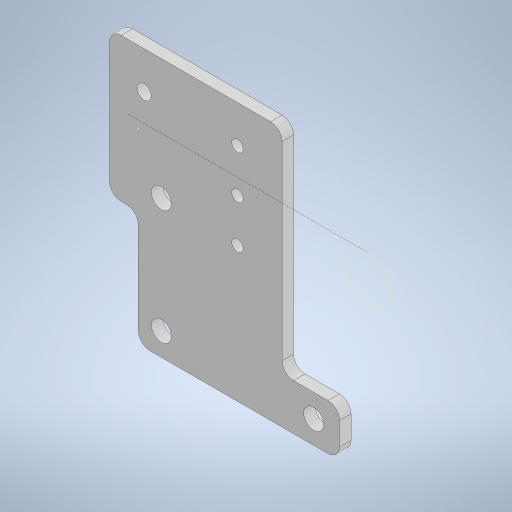
# Autodesk Inventor part: креп_центр_рейки
Saved by Autodesk Inventor 2023.1 (Build 271208000, 208)
## iProperties
Created: 2025-11-24
Part Number: креп_центр_рейки
Material: Типовые
Document SubType Name: Modeling
Designer: DELL
Density: 1 g/cm^3
Appearance: По умолчанию
Author: DELL
Autodesk Inventor part; units mm, degrees
ref_plane "YZ Plane" through (0, 0, 0) normal (1, 0, 0) x (0, 1, 0)
ref_plane "XZ Plane" through (0, 0, 0) normal (0, 1, 0) x (-1, 0, 0)
ref_plane "XY Plane" through (0, 0, 0) normal (0, 0, 1) x (1, 0, 0)
sketch "Эскиз1" plane through (0, 0, 0) normal (0, 0, 1) x (1, 0, 0)
  line L0 (4, 0) -> (50, 0)
  line L1 (70, -4) -> (70, -49)
  line L2 (66, -65) -> (4, -65)
  line L3 (0, -61) -> (0, -4)
  arc A0 (70, -4) -> (66, 0) centre (66, -4) ccw
  arc A1 (66, -65) -> (70, -61) centre (66, -61) ccw
  arc A2 (4, 0) -> (0, -4) centre (4, -4) ccw
  arc A3 (0, -61) -> (4, -65) centre (4, -61) ccw
  line L4 (-10, 25) -> (50, 25)
  line L5 (65, 25) -> (65, -25)
  line L6 (65, -25) -> (-10, -25)
  line L7 (-10, -25) -> (-10, 25)
  line L8 (-10, 25) -> (65, -25) construction
  line L9 (65, 25) -> (-10, -25) construction
  line L10 (70, -49) -> (50, -49)
  line L11 (50, -49) -> (50, 25)
  line L12 (70, -49) -> (70, -61)
  line L13 (65, 0) -> (66, 0)
  line L14 (50, 0) -> (65, 0)
  line L15 (50, 25) -> (65, 25)
  point P0 (0, 0)
  point P1 (70, -65)
  point P2 (70, 0)
  point P3 (27.5, 0)
  point P4 (5, 0)
  point P5 (65, 0)
  point P6 (50, -25)
  point P7 (0, -25)
  dimension "d0" = 70
  dimension "d1" = 65
  dimension "d2" = 4
  dimension "d23" = 75
  dimension "d24" = 50
  dimension "d44" = 20
  dimension "d46" = 16
  dimension "d47" = 5
  dimension "d48" = 25
  constraints: 32 end point, 14 tangent, 10 perpendicular, 8 parallel, 8 point on circle, 7 point on line, 6 horizontal, 4 centre point, 3 equal radius, 3 midpoint
  measures "d0" distance of point (0, 0) point (70, 0)
  measures "d1" distance of point (70, 0) point (70, -65)
  measures "d2" radius of A0
  measures "d23" distance of L5.end L6.end
  measures "d24" distance of L5.start L5.end
  measures "d44" distance of L1.end L10.end
  measures "d46" distance between parallel lines of L2 L10
  measures "d47" distance between parallel lines of L1 L5
  measures "d48" distance between parallel lines of L0 L4
extrude "Выдавливание1" add sketch "Эскиз1" along normal blind 4 contours A2 L3 L6 L7 L4 L11 L0 | L0 L11 L6 L3 A2 | L11 L10 L12 A1 L2 A3 L3 L6
sketch "Эскиз2" plane through (0, 0, 4) normal (0, 0, 1) x (1, 0, 0)
  circle A0 centre (61, -57) radius 3.5
  line L0 (4, -65) -> (66, -65) projected
  circle A1 centre (8, -57) radius 3.5
  line L1 (0, -25) -> (0, -61) projected
  circle A2 centre (61, -17) radius 3.5
  circle A3 centre (8, -17) radius 3.5
  line L2 (61, -17) -> (8, -17) construction
  line L3 (61, -17) -> (61, -57) construction
  line L4 (8, -57) -> (61, -57)
  circle A4 centre (54.5, 12) radius 2.5
  line L5 (54.5, 12) -> (54.5, -22.1685) construction
  circle A5 centre (2, 12) radius 2.5
  line L6 (70, -61) -> (70, -49) projected
  line L7 (-10, 25) -> (-10, -25) projected
  dimension "d5" = 7
  dimension "d6" = 8
  dimension "d8" = 7
  dimension "d9" = 8
  dimension "d10" = 8
  dimension "d13" = 7
  dimension "d16" = 7
  dimension "d19" = 53
  dimension "d20" = 53
  dimension "d21" = 40
  dimension "d22" = 40
  dimension "d26" = 5
  dimension "d27" = 29
  dimension "d28" = 6.5
  dimension "d29" = 5
  dimension "d43" = 29
  dimension "d51" = 12
  constraints: 8 end point, 6 centre point, 1 horizontal, 1 perpendicular, 1 vertical
  measures "d5" diameter of A0
  measures "d6" distance from line of L0 L3.end
  measures "d8" diameter of A1
  measures "d9" distance from line of L0 L4.start
  measures "d10" distance from line of L1 L4.start
  measures "d13" diameter of A2
  measures "d16" diameter of A3
  measures "d19" distance of L4.start L3.end
  measures "d20" distance of L2.end L2.start
  measures "d21" distance of L2.start L3.end
  measures "d22" distance of L4.start L2.end
  measures "d26" diameter of A4
  measures "d27" vertical distance of L5.start L2.start
  measures "d28" distance from line of L5 L2.start
  measures "d29" diameter of A5
  measures "d43" distance from line of L2 A5.centre
  measures "d51" distance from line of L7 A5.centre
extrude "Выдавливание2" cut sketch "Эскиз2" against normal blind 4
fillet "Сопряжение1" radius 4 1 edges at (-10, 25, 2)
sketch "Эскиз3" plane through (0, 0, 4) normal (0, 0, 1) x (1, 0, 0)
  circle A0 centre (2, 12) radius 2.5 construction
  line L0 (67, 12) -> (2, 12) construction
  line L1 (34.5, 12) -> (34.5, -39.6855) construction
  circle A1 centre (34.5, 12) radius 2
  circle A2 centre (34.5, -3) radius 2
  circle A3 centre (34.5, -18) radius 2
  line L2 (50, -49) -> (50, 25) projected
  point P0 (0, 0)
  dimension "d31" = 4
  dimension "d32" = 4
  dimension "d33" = 4
  dimension "d34" = 15
  dimension "d35" = 15
  dimension "d50" = 15.5
  constraints: 4 end point, 3 centre point, 2 point on line, 1 coincident, 1 horizontal, 1 midpoint, 1 vertical
  measures "d31" diameter of A1
  measures "d32" diameter of A2
  measures "d33" diameter of A3
  measures "d34" distance of A1.centre A2.centre
  measures "d35" distance of A2.centre A3.centre
  measures "d50" distance from line of L2 A2.centre
extrude "Выдавливание3" cut sketch "Эскиз3" against normal blind 10
fillet "Сопряжение3" radius 4 3 edges at (50, 25, 2) (50, -49, 2) (70, -49, 2)
sketch "Эскиз5" plane through (0, 0, 4) normal (0, 0, 1) x (1, 0, 0)
  circle A0 centre (79.889, -5.5) radius 8 construction
  line L0 (79.889, 2.5) -> (-3.7783, 2.5) construction
  point P0 (0, 0)
  constraints: 2 end point, 2 horizontal, 1 vertical alignment, 1 other
fillet "Сопряжение4" radius 4 2 edges at (0, -25, 2) (-10, -25, 2)
